rsp1Aholder (Autodesk Fusion 360 design; units mm, degrees)
Autodesk Fusion 360 part; units mm, degrees
note: some values were not read from the file. Chosen so that the rebuilt part matches the saved one: which face or edge a step refers to; which pieces of a blend or face edit are solid.
sketch "Sketch1" plane through (0, 0, 0) normal (1, 0, 0) x (0, 1, 0)
  line L0 (13, -20) -> (-13, -20)
  line L1 (-17.5, -15.8) -> (-17.5, 15.8)
  line L2 (12.9, 15.8) -> (12.9, -15.8)
  line L3 (13, -20) -> (-13, 20) construction
  line L4 (-13, -20) -> (13, 20) construction
  line L5 (-21.7, -15.8) -> (-21.7, 15.8)
  line L6 (-21.7, 15.8) -> (8.7, 15.8)
  line L7 (8.7, 15.8) -> (8.7, -15.8)
  line L8 (8.7, -15.8) -> (-21.7, -15.8)
  line L9 (-21.7, 15.8) -> (-17.5, 15.8)
  line L10 (8.7, 15.8) -> (12.9, 15.8)
  line L11 (-6.5, -15.8) -> (-34.8, -15.8)
  line L12 (-34.8, -15.8) -> (-34.8, -20)
  line L13 (-34.8, -20) -> (0, -20)
  line L14 (-4.4, -15.8) -> (26, -15.8)
  line L15 (26, -15.8) -> (26, -20)
  line L16 (26, -20) -> (0, -20)
  line L17 (-4.4, -15.8) -> (-4.4, 30)
  dimension "d38" = 13.1
  dimension "d39" = 13.1
  dimension "d40" = 4.2
  dimension "d41" = 4.2
  dimension "d42" = 13.1
  dimension "d44" = 13.1
  constraint horizontal L0
  constraint perpendicular L0 L1
  constraint coincident L3 origin
  constraint coincident L4 origin
  constraint perpendicular L1 L9
  constraint perpendicular L2 L10
  constraint parallel L0 L8
  constraint horizontal L11
  constraint vertical L12
  constraint horizontal L13
  constraint midpoint L8 L11.start
  constraint coincident L11 L1.start
  constraint coincident L14 L2.end
  constraint perpendicular L6 L17
  measures "d38" distance of L1 L17
  measures "d39" distance of L7 L17
  measures "d40" distance of L2 L7
  measures "d41" distance of L1 L5
  measures "d42" distance of L5.start L11.end
  measures "d44" distance of L2 L14.end
extrude "Extrude1" add sketch "Sketch1" along normal mid plane 44 contours L0 L8 L11 L12 L13 L14 L15 L16
extrude "Extrude2" add sketch "Sketch1" along normal mid plane 44 contours L2 L7 L10 L14 | L1 L5 L6 L8 L9 L11
extrude "Extrude3" add sketch "Sketch1" along normal mid plane 90 contours L0 L8 L11 L12 L13 L14 L15 L16
fillet "Fillet4" radius 9 4 edges at (22, 10.8, 15.8) (-22, 10.8, 15.8) (-22, -19.6, 15.8) (22, -19.6, 15.8)
sketch "Sketch3" plane through (0, 12.9, 0) normal (0, 1, 0) x (-1, 0, 0)
  arc A0 (22, 6.8) -> (13, 15.8) centre (13, 6.8) ccw
  line L0 (13, 15.8) -> (-13, 15.8)
  arc A1 (-13, 15.8) -> (-22, 6.8) centre (-13, 6.8) ccw
  line L1 (-22, 6.8) -> (-22, -15.8)
  line L2 (-22, -15.8) -> (22, -15.8)
  line L3 (22, -15.8) -> (22, 6.8)
  line L4 (-19.4275, -5.5539) -> (-19.4275, 2.4461)
  line L5 (-19.4275, 2.4461) -> (-18.3688, 2.4461)
  line L6 (-18.3688, 2.4461) -> (-18.3688, -5.5539)
  line L7 (-18.3688, -5.5539) -> (-19.4275, -5.5539)
  line L8 (-16.5134, -5.5539) -> (-16.5134, 2.4461)
  line L9 (-16.5134, 2.4461) -> (-15.4275, 2.4461)
  line L10 (-15.4275, 2.4461) -> (-11.2256, -3.8349)
  line L11 (-11.2256, -3.8349) -> (-11.2256, 2.4461)
  line L12 (-11.2256, 2.4461) -> (-10.2106, 2.4461)
  line L13 (-10.2106, 2.4461) -> (-10.2106, -5.5539)
  line L14 (-10.2106, -5.5539) -> (-11.2965, -5.5539)
  line L15 (-11.2965, -5.5539) -> (-15.4984, 0.7326)
  line L16 (-15.4984, 0.7326) -> (-15.4984, -5.5539)
  line L17 (-15.4984, -5.5539) -> (-16.5134, -5.5539)
  line L18 (-8.8245, -3.442) -> (-7.8422, -3.311)
  spline S0 degree 3 poles (-7.8422, -3.311) (-7.7856, -3.5603) (-7.6842, -4.0067) (-7.3945, -4.3588) (-7.2665, -4.5143) knots 0 0 0 0 0.075375 0.135022 0.135022 0.135022 0.135022
  spline S1 degree 3 poles (-7.2665, -4.5143) (-7.122, -4.6217) (-6.8278, -4.8403) (-6.4621, -4.8684) (-6.276, -4.8826) knots 0 0 0 0 0.052879 0.107616 0.107616 0.107616 0.107616
  spline S2 degree 3 poles (-6.276, -4.8826) (-6.0545, -4.8632) (-5.6144, -4.8244) (-5.2744, -4.5425) (-5.1055, -4.4024) knots 0 0 0 0 0.065033 0.129227 0.129227 0.129227 0.129227
  spline S3 degree 3 poles (-5.1055, -4.4024) (-4.9662, -4.2313) (-4.684, -3.8845) (-4.6469, -3.4386) (-4.628, -3.2128) knots 0 0 0 0 0.064589 0.130884 0.130884 0.130884 0.130884
  spline S4 degree 3 poles (-4.628, -3.2128) (-4.6447, -2.9989) (-4.6772, -2.5808) (-4.9411, -2.2557) (-5.07, -2.0968) knots 0 0 0 0 0.062714 0.122592 0.122592 0.122592 0.122592
  spline S5 degree 3 poles (-5.07, -2.0968) (-5.2301, -1.9687) (-5.5586, -1.7059) (-5.9788, -1.6739) (-6.1942, -1.6575) knots 0 0 0 0 0.06005 0.123222 0.123222 0.123222 0.123222
  spline S6 degree 3 poles (-6.1942, -1.6575) (-6.2988, -1.6638) (-6.5331, -1.6777) (-6.761, -1.735) (-6.8872, -1.7667) knots 0 0 0 0 0.03136 0.070293 0.070293 0.070293 0.070293
  line L19 (-6.8872, -1.7667) -> (-6.7781, -0.9045)
  spline S7 degree 3 poles (-6.7781, -0.9045) (-6.7486, -0.9076) (-6.6959, -0.9133) (-6.643, -0.9147) (-6.6198, -0.9154) knots 0 0 0 0 0.008905 0.015868 0.015868 0.015868 0.015868
  spline S8 degree 3 poles (-6.6198, -0.9154) (-6.4169, -0.9024) (-6.016, -0.8768) (-5.6641, -0.6835) (-5.4902, -0.588) knots 0 0 0 0 0.060177 0.118901 0.118901 0.118901 0.118901
  spline S9 degree 3 poles (-5.4902, -0.588) (-5.3439, -0.4599) (-5.0393, -0.1934) (-5.0056, 0.2113) (-4.9882, 0.4216) knots 0 0 0 0 0.056117 0.116775 0.116775 0.116775 0.116775
  spline S10 degree 3 poles (-4.9882, 0.4216) (-5.0024, 0.5929) (-5.0303, 0.93) (-5.2472, 1.1891) (-5.3538, 1.3165) knots 0 0 0 0 0.050225 0.098812 0.098812 0.098812 0.098812
  spline S11 degree 3 poles (-5.3538, 1.3165) (-5.4877, 1.42) (-5.7655, 1.6344) (-6.1163, 1.6587) (-6.2979, 1.6712) knots 0 0 0 0 0.049617 0.102885 0.102885 0.102885 0.102885
  spline S12 degree 3 poles (-6.2979, 1.6712) (-6.4793, 1.6578) (-6.8335, 1.6314) (-7.1153, 1.4161) (-7.2528, 1.3111) knots 0 0 0 0 0.05329 0.104049 0.104049 0.104049 0.104049
  spline S13 degree 3 poles (-7.2528, 1.3111) (-7.37, 1.1669) (-7.6269, 0.8508) (-7.7027, 0.4491) (-7.744, 0.2306) knots 0 0 0 0 0.054876 0.120353 0.120353 0.120353 0.120353
  line L20 (-7.744, 0.2306) -> (-8.7262, 0.4052)
  spline S14 degree 3 poles (-8.7262, 0.4052) (-8.6528, 0.7109) (-8.5128, 1.2937) (-8.1027, 1.729) (-7.9077, 1.9359) knots 0 0 0 0 0.092474 0.176282 0.176282 0.176282 0.176282
  spline S15 degree 3 poles (-7.9077, 1.9359) (-7.6768, 2.0942) (-7.1987, 2.4221) (-6.6193, 2.4595) (-6.3197, 2.4789) knots 0 0 0 0 0.082391 0.170618 0.170618 0.170618 0.170618
  spline S16 degree 3 poles (-6.3197, 2.4789) (-6.1071, 2.4679) (-5.6882, 2.4462) (-5.3033, 2.2798) (-5.1137, 2.1978) knots 0 0 0 0 0.063283 0.12472 0.12472 0.12472 0.12472
  spline S17 degree 3 poles (-5.1137, 2.1978) (-4.942, 2.0976) (-4.6063, 1.9017) (-4.3808, 1.5855) (-4.2706, 1.4311) knots 0 0 0 0 0.058898 0.115119 0.115119 0.115119 0.115119
  spline S18 degree 3 poles (-4.2706, 1.4311) (-4.1854, 1.2677) (-4.0168, 0.9439) (-3.9913, 0.5799) (-3.9786, 0.3998) knots 0 0 0 0 0.054647 0.108216 0.108216 0.108216 0.108216
  spline S19 degree 3 poles (-3.9786, 0.3998) (-3.99, 0.2312) (-4.0126, -0.1042) (-4.1758, -0.3981) (-4.2569, -0.5443) knots 0 0 0 0 0.050009 0.099509 0.099509 0.099509 0.099509
  spline S20 degree 3 poles (-4.2569, -0.5443) (-4.3646, -0.6806) (-4.5897, -0.9657) (-4.9125, -1.1334) (-5.081, -1.221) knots 0 0 0 0 0.051483 0.107709 0.107709 0.107709 0.107709
  spline S21 degree 3 poles (-5.081, -1.221) (-4.8599, -1.2873) (-4.4314, -1.416) (-4.1263, -1.7424) (-3.9786, -1.9004) knots 0 0 0 0 0.067869 0.131566 0.131566 0.131566 0.131566
  spline S22 degree 3 poles (-3.9786, -1.9004) (-3.8641, -2.0888) (-3.6235, -2.4846) (-3.5987, -2.9481) (-3.5857, -3.191) knots 0 0 0 0 0.0651 0.136786 0.136786 0.136786 0.136786
  spline S23 degree 3 poles (-3.5857, -3.191) (-3.6178, -3.5272) (-3.6822, -4.201) (-4.1269, -4.7115) (-4.3497, -4.9672) knots 0 0 0 0 0.09866 0.197741 0.197741 0.197741 0.197741
  spline S24 degree 3 poles (-4.3497, -4.9672) (-4.6264, -5.1797) (-5.1958, -5.6168) (-5.9129, -5.669) (-6.2815, -5.6957) knots 0 0 0 0 0.102306 0.210535 0.210535 0.210535 0.210535
  spline S25 degree 3 poles (-6.2815, -5.6957) (-6.6136, -5.6731) (-7.2571, -5.6294) (-7.7783, -5.2512) (-8.0305, -5.0682) knots 0 0 0 0 0.097653 0.189193 0.189193 0.189193 0.189193
  spline S26 degree 3 poles (-8.0305, -5.0682) (-8.2378, -4.8405) (-8.6604, -4.3763) (-8.7691, -3.7573) (-8.8245, -3.442) knots 0 0 0 0 0.090411 0.18432 0.18432 0.18432 0.18432
  line L21 (-3.0946, -5.5539) -> (-0.0223, 2.4461)
  line L22 (-0.0223, 2.4461) -> (1.1182, 2.4461)
  line L23 (1.1182, 2.4461) -> (4.3924, -5.5539)
  line L24 (4.3924, -5.5539) -> (3.1864, -5.5539)
  line L25 (3.1864, -5.5539) -> (2.2533, -3.1309)
  line L26 (2.2533, -3.1309) -> (-1.0919, -3.1309)
  line L27 (-1.0919, -3.1309) -> (-1.9704, -5.5539)
  line L28 (-1.9704, -5.5539) -> (-3.0946, -5.5539)
  line L29 (-0.7863, -2.2687) -> (1.9259, -2.2687)
  line L30 (1.9259, -2.2687) -> (1.0909, -0.0532)
  spline S27 degree 3 poles (1.0909, -0.0532) (0.9765, 0.2522) (0.7714, 0.7997) (0.5995, 1.3585) (0.5234, 1.6058) knots 0 0 0 0 0.097791 0.175368 0.175368 0.175368 0.175368
  spline S28 degree 3 poles (0.5234, 1.6058) (0.4669, 1.3488) (0.3531, 0.8311) (0.1797, 0.3301) (0.0923, 0.0778) knots 0 0 0 0 0.078852 0.158883 0.158883 0.158883 0.158883
  line L31 (0.0923, 0.0778) -> (-0.7863, -2.2687)
  spline S29 degree 3 poles (11.301, -4.6971) (11.5328, -4.8514) (11.9642, -5.1386) (12.4398, -5.3441) (12.6598, -5.4393) knots 0 0 0 0 0.083325 0.155103 0.155103 0.155103 0.155103
  line L32 (12.6598, -5.4393) -> (12.3488, -6.176)
  spline S30 degree 3 poles (12.3488, -6.176) (12.0559, -6.0527) (11.4434, -5.795) (10.9088, -5.3999) (10.6298, -5.1937) knots 0 0 0 0 0.09497 0.19861 0.19861 0.19861 0.19861
  spline S31 degree 3 poles (10.6298, -5.1937) (10.3231, -5.3385) (9.701, -5.6323) (9.0138, -5.6708) (8.6653, -5.6903) knots 0 0 0 0 0.100727 0.204338 0.204338 0.204338 0.204338
  spline S32 degree 3 poles (8.6653, -5.6903) (8.3139, -5.6698) (7.6213, -5.6293) (7.001, -5.3192) (6.6953, -5.1664) knots 0 0 0 0 0.104372 0.205747 0.205747 0.205747 0.205747
  spline S33 degree 3 poles (6.6953, -5.1664) (6.4169, -4.9727) (5.855, -4.5816) (5.5085, -3.991) (5.3338, -3.693) knots 0 0 0 0 0.10047 0.202755 0.202755 0.202755 0.202755
  spline S34 degree 3 poles (5.3338, -3.693) (5.1945, -3.361) (4.9077, -2.6769) (4.8737, -1.9355) (4.8563, -1.5539) knots 0 0 0 0 0.107119 0.220708 0.220708 0.220708 0.220708
  spline S35 degree 3 poles (4.8563, -1.5539) (4.8744, -1.1719) (4.9098, -0.4253) (5.1965, 0.2647) (5.3365, 0.6017) knots 0 0 0 0 0.113732 0.222334 0.222334 0.222334 0.222334
  spline S36 degree 3 poles (5.3365, 0.6017) (5.5111, 0.9047) (5.855, 1.5015) (6.4236, 1.8896) (6.7035, 2.0805) knots 0 0 0 0 0.103453 0.203709 0.203709 0.203709 0.203709
  spline S37 degree 3 poles (6.7035, 2.0805) (7.0111, 2.2285) (7.6381, 2.5302) (8.3331, 2.5685) (8.6871, 2.588) knots 0 0 0 0 0.101348 0.20655 0.20655 0.20655 0.20655
  spline S38 degree 3 poles (8.6871, 2.588) (9.0445, 2.5677) (9.7464, 2.5279) (10.3755, 2.215) (10.6844, 2.0614) knots 0 0 0 0 0.10614 0.208475 0.208475 0.208475 0.208475
  spline S39 degree 3 poles (10.6844, 2.0614) (10.9637, 1.8675) (11.5254, 1.4775) (11.8682, 0.8856) (12.0405, 0.588) knots 0 0 0 0 0.100661 0.202449 0.202449 0.202449 0.202449
  spline S40 degree 3 poles (12.0405, 0.588) (12.1765, 0.2565) (12.4573, -0.4278) (12.4901, -1.1672) (12.507, -1.5484) knots 0 0 0 0 0.106654 0.220148 0.220148 0.220148 0.220148
  spline S41 degree 3 poles (12.507, -1.5484) (12.4967, -1.8636) (12.4768, -2.4695) (12.2944, -3.0474) (12.2069, -3.3247) knots 0 0 0 0 0.094092 0.180895 0.180895 0.180895 0.180895
  spline S42 degree 3 poles (12.2069, -3.3247) (12.0942, -3.5789) (11.869, -4.087) (11.4903, -4.4938) (11.301, -4.6971) knots 0 0 0 0 0.082796 0.165469 0.165469 0.165469 0.165469
  spline S43 degree 3 poles (8.9709, -3.3438) (9.2574, -3.435) (9.8028, -3.6087) (10.2637, -3.9471) (10.4825, -4.1077) knots 0 0 0 0 0.089515 0.170375 0.170375 0.170375 0.170375
  spline S44 degree 3 poles (10.4825, -4.1077) (10.7541, -3.7674) (11.348, -3.0233) (11.3918, -2.0672) (11.4156, -1.5484) knots 0 0 0 0 0.127478 0.278675 0.278675 0.278675 0.278675
  spline S45 degree 3 poles (11.4156, -1.5484) (11.4049, -1.2417) (11.3845, -0.6581) (11.1817, -0.1109) (11.0855, 0.1487) knots 0 0 0 0 0.091369 0.17389 0.17389 0.17389 0.17389
  spline S46 degree 3 poles (11.0855, 0.1487) (10.9644, 0.376) (10.726, 0.8236) (10.3196, 1.1265) (10.1196, 1.2756) knots 0 0 0 0 0.076211 0.150065 0.150065 0.150065 0.150065
  spline S47 degree 3 poles (10.1196, 1.2756) (9.8994, 1.3926) (9.4531, 1.6298) (8.9484, 1.6609) (8.6926, 1.6767) knots 0 0 0 0 0.073865 0.149769 0.149769 0.149769 0.149769
  spline S48 degree 3 poles (8.6926, 1.6767) (8.3166, 1.6449) (7.5754, 1.5823) (7.0078, 1.1027) (6.7281, 0.8663) knots 0 0 0 0 0.1102 0.217256 0.217256 0.217256 0.217256
  spline S49 degree 3 poles (6.7281, 0.8663) (6.501, 0.5406) (5.9972, -0.1823) (5.9653, -1.0675) (5.9477, -1.5539) knots 0 0 0 0 0.116752 0.259091 0.259091 0.259091 0.259091
  spline S50 degree 3 poles (5.9477, -1.5539) (5.9671, -2.0289) (6.0027, -2.9031) (6.4951, -3.6215) (6.7199, -3.9495) knots 0 0 0 0 0.139271 0.256249 0.256249 0.256249 0.256249
  spline S51 degree 3 poles (6.7199, -3.9495) (6.9981, -4.193) (7.5633, -4.6876) (8.3123, -4.7518) (8.6926, -4.7844) knots 0 0 0 0 0.107946 0.219265 0.219265 0.219265 0.219265
  spline S52 degree 3 poles (8.6926, -4.7844) (8.8781, -4.7759) (9.2455, -4.7591) (9.5911, -4.6337) (9.7622, -4.5716) knots 0 0 0 0 0.055372 0.109616 0.109616 0.109616 0.109616
  spline S53 degree 3 poles (9.7622, -4.5716) (9.5953, -4.4723) (9.2652, -4.2756) (8.8967, -4.167) (8.7144, -4.1132) knots 0 0 0 0 0.05799 0.114765 0.114765 0.114765 0.114765
  line L33 (8.7144, -4.1132) -> (8.9709, -3.3438)
  line L34 (13.8877, -5.5539) -> (13.8877, 2.4461)
  line L35 (13.8877, 2.4461) -> (14.9463, 2.4461)
  line L36 (14.9463, 2.4461) -> (14.9463, -1.5211)
  line L37 (14.9463, -1.5211) -> (18.919, 2.4461)
  line L38 (18.919, 2.4461) -> (20.3542, 2.4461)
  line L39 (20.3542, 2.4461) -> (16.9982, -0.7953)
  line L40 (16.9982, -0.7953) -> (20.5016, -5.5539)
  line L41 (20.5016, -5.5539) -> (19.1046, -5.5539)
  line L42 (19.1046, -5.5539) -> (16.256, -1.5047)
  line L43 (16.256, -1.5047) -> (14.9463, -2.7817)
  line L44 (14.9463, -2.7817) -> (14.9463, -5.5539)
  line L45 (14.9463, -5.5539) -> (13.8877, -5.5539)
extrude "Extrude5" cut sketch "Sketch3" against normal blind 1.2 contours L4 L5 L6 L7 | L8 L9 L10 L11 L12 L13 L14 L15 L16 L17 | L18 S0 S1 S2 S3 S4 S5 S6 L19 S7 S8 S9 S10 S11 S12 S13 L20 S14 S15 S16 S17 S18 S19 S20 S21 S22 S23 S24 S25 S26 | L21 L22 L23 L24 L25 L26 L27 L28 | S29 L32 S30 S31 S32 S33 S34 S35 S36 S37 S38 S39 S40 S41 S42 | L34 L35 L36 L37 L38 L39 L40 L41 L42 L43 L44 L45
fillet "Fillet8" radius 1.5 10 edges at (22, 12.9, -4.5) (19.364, 12.9, 13.164) (0, 12.9, 15.8) (-19.364, 12.9, 13.164) (-22, 12.9, -4.5) (-22, -21.7, -4.5) (-19.364, -21.7, 13.164) (0, -21.7, 15.8) (19.364, -21.7, 13.164) (22, -21.7, -4.5)
fillet "Fillet9" radius 1.5 14 edges at (0, -21.7, -15.8) (-21.5629, -21.2629, -15.8) (21.5629, -21.2629, -15.8) (-22, -18.8537, -15.8) (22, -18.8537, -15.8) (-45, -4.4, -15.8) (0, 26, -15.8) (45, -4.4, -15.8) (0, -34.8, -15.8) (22, 10.0538, -15.8) (21.5629, 12.4629, -15.8) (0, 12.9, -15.8) (-22, 10.0538, -15.8) (-21.5629, 12.4629, -15.8)
fillet "Fillet10" radius 2.5 2 edges at (0, -17.5, -15.8) (0, 8.7, -15.8)
fillet "Fillet11" radius 20.5 8 edges at (45, 26, -18.65) (44.5607, 25.5607, -16.2393) (-45, 26, -18.65) (-44.5607, 25.5607, -16.2393) (45, -34.8, -18.65) (44.5607, -34.3607, -16.2393) (-44.5607, -34.3607, -16.2393) (-45, -34.8, -18.65)
